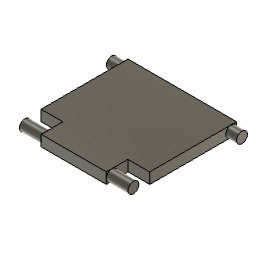
_clamp top.46419cef-eac4-46b9-a695-fc1142d0df38 (Autodesk Fusion 360 design; units mm, degrees)
Autodesk Fusion 360 part; units mm, degrees
sketch "Sketch1" plane through (0, 0, 0) normal (0, 0, 1) x (1, 0, 0)
  line L0 (0, 0) -> (30, 0)
  line L1 (30, 0) -> (30, 50)
  line L2 (30, 50) -> (0, 50)
  line L3 (0, 50) -> (0, 0)
  dimension "d1" = 30
  dimension "d2" = 50
  constraint horizontal L0
  constraint vertical L1
  constraint horizontal L2
  constraint vertical L3
  constraint coincident L0.start L3.end
  measures "d1" distance of L0.start L0.end
  measures "d2" distance of L0.start L2.end
extrude "Extrude1" add sketch "Sketch1" along normal blind 5
sketch "Sketch3" plane through (30, 0, 0) normal (1, 0, 0) x (0, 1, 0)
  line L0 (0, 0) -> (50, 0)
  line L1 (50, 0) -> (50, 5)
  line L2 (50, 5) -> (0, 5)
  line L3 (0, 5) -> (0, 0)
  line L4 (50, 5) -> (10, 5)
  line L5 (10, 5) -> (10, 0)
  line L6 (10, 0) -> (50, 0)
  line L7 (50, 0) -> (50, 5)
  dimension "d9" = 40
  dimension "d10" = 5
  constraint horizontal L4
  constraint vertical L5
  constraint horizontal L6
  constraint vertical L7
  constraint coincident L1.end L2.start
  measures "d9" distance of L1.end L4.end
  measures "d10" distance of L1.end L0.end
extrude "Extrude3" add sketch "Sketch3" along normal blind 10 contours L0 L1 L2 L4 L5 L6 L7
sketch "Sketch4" plane through (0, 0, 0) normal (-1, 0, 0) x (0, -1, 0)
  line L0 (-50, 0) -> (0, 0)
  line L1 (0, 0) -> (0, 5)
  line L2 (0, 5) -> (-50, 5)
  line L3 (-50, 5) -> (-50, 0)
  line L4 (-50, 5) -> (-10, 5)
  line L5 (-10, 5) -> (-10, 0)
  line L6 (-10, 0) -> (-50, 0)
  line L7 (-50, 0) -> (-50, 5)
  dimension "d13" = 40
  dimension "d14" = 5
  constraint horizontal L4
  constraint vertical L5
  constraint horizontal L6
  constraint vertical L7
  constraint coincident L2.end L3.start
  measures "d13" distance of L2.end L4.end
  measures "d14" distance of L2.end L0.start
extrude "Extrude4" add sketch "Sketch4" along normal blind 10 contours L0 L2 L3 L4 L5 L6 L7
sketch "Sketch5" plane through (0, 0, 0) normal (-1, 0, 0) x (0, -1, 0)
  line L0 (-10, 5) -> (-10, 0)
  line L1 (-10, 0) -> (0, 0)
  line L2 (0, 0) -> (0, 5)
  line L3 (0, 5) -> (-10, 5)
  circle A0 centre (-2.5, 2.5) radius 2.5
  dimension "d17" = 5
  measures "d17" diameter of A0
extrude "Extrude5" add sketch "Sketch5" along normal blind 10 contours A0
sketch "Sketch6" plane through (30, 0, 0) normal (1, 0, 0) x (0, 1, 0)
  line L0 (10, 0) -> (10, 5)
  line L1 (10, 5) -> (0, 5)
  line L2 (0, 5) -> (0, 0)
  line L3 (0, 0) -> (10, 0)
  circle A0 centre (2.5, 2.5) radius 2.5
  dimension "d20" = 5
  measures "d20" diameter of A0
extrude "Extrude6" add sketch "Sketch6" along normal blind 10 contours A0
sketch "Sketch7" plane through (40, 0, 0) normal (1, 0, 0) x (0, 1, 0)
  line L0 (50, 0) -> (50, 5)
  line L1 (50, 5) -> (10, 5)
  line L2 (10, 5) -> (10, 0)
  line L3 (10, 0) -> (50, 0)
  circle A0 centre (47.5, 2.5) radius 2.5
  dimension "d23" = 5
  measures "d23" diameter of A0
extrude "Extrude7" add sketch "Sketch7" along normal blind 5 contours A0
sketch "Sketch8" plane through (-10, 0, 0) normal (-1, 0, 0) x (0, -1, 0)
  line L0 (-50, 0) -> (-10, 0)
  line L1 (-10, 0) -> (-10, 5)
  line L2 (-10, 5) -> (-50, 5)
  line L3 (-50, 5) -> (-50, 0)
  circle A0 centre (-47.5, 2.5) radius 2.5
  dimension "d26" = 5
  measures "d26" diameter of A0
extrude "Extrude8" add sketch "Sketch8" along normal blind 5 contours A0
